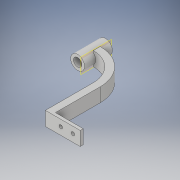
# Autodesk Inventor part: Base
Saved by Autodesk Inventor 2019 (Build 230136000, 136)
## iProperties
Created: 2019-05-09
Part Number: Base
Material: Generic
Document SubType Name: Modeling
Designer: riphipps21
Density: 1 g/cm^3
Appearance: Default
Author: riphipps21
Autodesk Inventor part; units mm, degrees
ref_plane "XZ Plane" through (0, 0, 0) normal (0, 1, 0) x (-1, 0, 0)
ref_plane "XY Plane" through (0, 0, 0) normal (0, 0, 1) x (1, 0, 0)
sketch "Sketch1" plane through (0, 0, 0) normal (0, 0, 1) x (1, 0, 0)
  point P0 (0, 0)
sketch "Sketch2" plane through (0, 0, 0) normal (0, 0, 1) x (1, 0, 0)
  circle A0 centre (1.095, 0) radius 3.175
  point P0 (0, 0)
  constraints: 1 centre point
extrude "Extrusion1" add sketch "Sketch2" along normal blind 12.7
sketch "Sketch3" plane through (1.095, 0, 12.7) normal (0, 0, 1) x (1, 0, 0)
  point P0 (-1.095, 0)
  point P1 (0.0374, 0.0562)
hole "Hole1" at (1.1325, 0.0562, 12.7) direction (0, 0, -1) diameter 3.81 end through all
ref_plane "Work Plane1" through (3.175, 0, 0) normal (1, 0, 0) x (0, 1, 0)
sketch "Sketch4" plane through (3.175, 0, 0) normal (1, 0, 0) x (0, 1, 0)
  line L0 (3.175, 0) -> (3.175, 12.7) projected
  line L1 (3.175, 7.62) -> (-3.175, 7.62)
  line L2 (-3.175, 7.62) -> (-3.175, 4.445)
  line L3 (-3.175, 4.445) -> (3.175, 4.445)
  line L4 (3.175, 4.445) -> (3.175, 7.62)
  line L5 (3.175, 12.7) -> (-3.175, 12.7) projected
  line L6 (-3.175, 0) -> (-3.175, 12.7) projected
  point P0 (0, 0)
  dimension "d11" = 3.175
  dimension "d12" = 5.08
  constraints: 8 end point, 2 parallel, 1 collinear, 1 horizontal, 1 perpendicular, 1 point on line
  measures "d11" distance between parallel lines of L1 L3
  measures "d12" distance between parallel lines of L1 L5
sketch "Sketch5" plane through (0, 0, 0) normal (0, 1, 0) x (-1, 0, 0)
  line L0 (-3.175, 0) -> (-3.175, 12.7) projected
  arc A0 (-15.875, 20.32) -> (-3.175, 7.62) centre (-3.175, 20.32) ccw
  line L1 (-3.175, 20.32) -> (-15.875, 20.32) construction
  line L2 (2.08, 12.7) -> (-4.27, 12.7) projected
  line L3 (-15.875, 20.32) -> (-15.875, 42.189)
  point P0 (0, 0)
  dimension "d13" = 12.7
  dimension "d14" = 5.08
  dimension "d15" = 0
  constraints: 4 end point, 2 point on circle, 1 centre point, 1 horizontal, 1 point on line, 1 vertical
  measures "d13" radius of A0
  measures "d14" distance from line of L2 A0.end
  measures "d15" distance from line of L1.start L0
sweep "Sweep1" add profiles "Sketch4" path "Sketch5" path curves A0 L3 contours L3 L2 L1 L0
sketch "Sketch6" plane through (19.05, -3.175, 20.32) normal (1, 0, 0) x (0, 0, -1)
  line L0 (-21.869, 0) -> (-21.869, 6.35) projected
  line L1 (0, 0) -> (-21.869, 0) projected
  line L2 (-21.869, 6.35) -> (-20.4611, 6.35)
  line L3 (-20.4611, 6.35) -> (-20.4611, 0)
  line L4 (-20.4611, 0) -> (-21.869, 0)
  line L5 (-21.869, 0) -> (-21.869, 6.35)
  point P0 (20.32, 3.175)
  constraints: 8 end point, 2 parallel, 1 horizontal, 1 perpendicular, 1 point on line
extrude "Extrusion2" add sketch "Sketch6" along normal blind 12.7
sketch "Sketch7" plane through (19.05, -3.175, 40.7811) normal (0, 0, -1) x (-1, 0, 0)
  circle A0 centre (-9.4194, 3.417) radius 0.7938
  circle A1 centre (-3.8794, 3.417) radius 0.7938
  point P0 (19.05, 3.175)
  constraints: 2 centre point
extrude "Extrusion3" cut sketch "Sketch7" against normal blind 12.7
body "Solid1"
